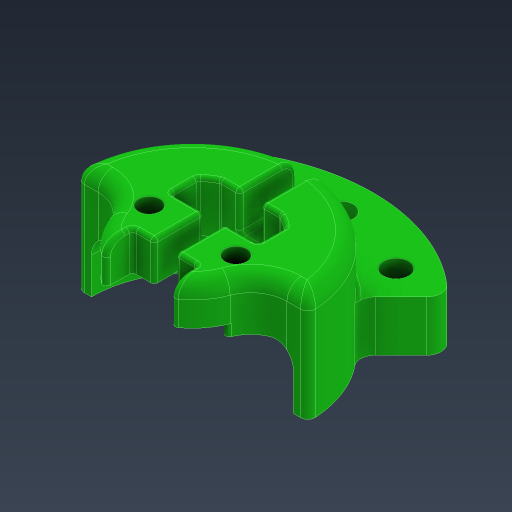
# Autodesk Inventor part: Крепление_энкодера
Saved by Autodesk Inventor 2023.2 (Build 272271030, 271C)
## iProperties
Created: 2026-01-03
Part Number: Крепление_энкодера
Material: Типовые
Document SubType Name: Modeling
Designer: Олег Коноваленко
Density: 1 g/cm^3
Appearance: Темно-зеленый
Author: Олег Коноваленко
Autodesk Inventor part; units mm, degrees
ref_plane "YZ Plane" through (0, 0, 0) normal (1, 0, 0) x (0, 1, 0)
ref_plane "XZ Plane" through (0, 0, 0) normal (0, 1, 0) x (-1, 0, 0)
ref_plane "XY Plane" through (0, 0, 0) normal (0, 0, 1) x (1, 0, 0)
sketch "Эскиз1" plane through (0, 0, 0) normal (0, 1, 0) x (-1, 0, 0)
  arc A0 (-14, 0) -> (14, 0) centre (0, 0) ccw
  arc A1 (-16, 0) -> (16, 0) centre (0, 0) ccw
  line L0 (-22.4, 0) -> (22.4, 0) projected
  dimension "d0" = 14
  dimension "d1" = 16
  constraints: 4 point on circle, 2 centre point, 2 point on line, 1 coincident
  measures "d0" radius of A0
  measures "d1" radius of A1
extrude "Выдавливание1" add sketch "Эскиз1" along normal blind 3 and the other way blind 5 contours A0 L0 A1
sketch "Эскиз2" plane through (0, 3, 0) normal (0, 1, 0) x (1, 0, 0)
  arc A0 (14, 0) -> (-14, 0) centre (0, 0) ccw projected
  circle A1 centre (0, 0) radius 9
  arc A2 (16, 0) -> (-16, 0) centre (0, 0) ccw projected
  line L0 (22.4, 0) -> (-22.4, 0) projected
  point P0 (-9, 0)
  point P1 (9, 0)
  dimension "d7" = 18
  constraints: 1 centre point, 1 coincident
  measures "d7" diameter of A1
extrude "Выдавливание2" add sketch "Эскиз2" along normal blind 7
fillet "Сопряжение2" radius 5 2 edges at (-9, 6.5, 0) (9, 6.5, 0)
fillet "Сопряжение3" radius 2 6 edges at (0, 10, -16) (10.242, 10, 0.8812) (14.5383, 10, 0) (-10.242, 10, 0.8812) (-14.5383, 10, 0) (0, 10, 9)
sketch "Эскиз3" plane through (0, 3, 0) normal (0, -1, 0) x (1, 0, 0)
  circle A0 centre (6, 0) radius 1.1 projected
  circle A1 centre (-6, 0) radius 1.1 projected
  circle A2 centre (-6, 0) radius 1.5
  circle A3 centre (6, 0) radius 1.5
  point P0 (0, 0)
  dimension "d12" = 3
  constraints: 2 centre point, 2 coincident, 1 equal radius
  measures "d12" diameter of A2
extrude "Выдавливание3" cut sketch "Эскиз3" against normal up to next contours A0 | A1 | A2 | A3
sketch "Эскиз4" plane through (0, 3, 0) normal (0, -1, 0) x (1, 0, 0)
  arc A0 (-7.5, -4.9749) -> (-4.1231, -8) centre (0, 0) ccw projected
  line L0 (4.1231, -8) -> (-4.1231, -8) projected
  arc A1 (4.1231, -8) -> (7.5, -4.9749) centre (0, 0) ccw projected
  line L1 (7.5, -4.9749) -> (7.5, 4.9749) projected
  arc A2 (7.5, 4.9749) -> (-7.5, 4.9749) centre (0, 0) ccw projected
  line L2 (-7.5, -4.9749) -> (-7.5, 4.9749) projected
extrude "Выдавливание4" cut sketch "Эскиз4" against normal blind 1.6
fillet "Сопряжение4" radius 0.5 2 edges at (-7.5, 3.8, 4.9749) (7.5, 3.8, 4.9749)
sketch "Эскиз5" plane through (0, -5, 0) normal (0, -1, 0) x (1, 0, 0)
  arc A0 (-17.6777, -17.6777) -> (17.6777, -17.6777) centre (0, 0) ccw
  line L0 (0, 5) -> (0, -30) construction
  line L1 (17.6777, -17.6777) -> (11.3137, -11.3137)
  arc A1 (-16, 0) -> (16, 0) centre (0, 0) ccw projected
  line L2 (-17.6777, -17.6777) -> (-11.3137, -11.3137)
  arc A2 (-14.4957, -14.4957) -> (14.4957, -14.4957) centre (0, 0) ccw construction
  circle A3 centre (10.6777, -17.4996) radius 1.75
  circle A4 centre (-10.6777, -17.4996) radius 1.75
  circle A5 centre (0, -20.5) radius 1.75
  point P0 (0, -25)
  dimension "d18" = 25
  dimension "d19" = 3.5
  dimension "d20" = 7
  dimension "d21" = 7
  constraints: 11 point on circle, 5 centre point, 4 end point, 2 coincident, 2 equal radius, 2 line through centre, 2 midpoint, 1 perpendicular, 1 point on line
  measures "d18" radius of A0
  measures "d19" diameter of A3
  measures "d20" horizontal distance of A3.centre L1.start
  measures "d21" horizontal distance of L2.start A4.centre
extrude "Выдавливание5" add sketch "Эскиз5" against normal blind 7
fillet "Сопряжение5" radius 2 4 edges at (11.3137, -1.5, -11.3137) (-11.3137, -1.5, -11.3137) (-17.6777, -1.5, -17.6777) (17.6777, -1.5, -17.6777)
sketch "Эскиз6" plane through (0, 4.6, 0) normal (0, -1, 0) x (1, 0, 0)
  line L0 (0, 15.8) -> (0, -31.8) construction
  line L1 (-4.5, 7.7942) -> (4.5, 7.7942) construction
  line L2 (4.5, 7.7942) -> (4.5, 3.7942)
  line L3 (4.5, 3.7942) -> (-4.5, 3.7942)
  line L4 (-4.5, 3.7942) -> (-4.5, 7.7942)
  line L5 (-4.5, 7.7942) -> (4.5, 3.7942) construction
  line L6 (4.5, 7.7942) -> (-4.5, 3.7942) construction
  arc A0 (8.4064, 3.2143) -> (-8.4064, 3.2143) centre (0, 0) ccw projected
  point P0 (0, 5.7942)
  point P1 (-4.5, 7.7942)
  dimension "d25" = 4
  dimension "d26" = 9
  constraints: 12 end point, 2 midpoint, 2 parallel, 1 horizontal, 1 perpendicular, 1 point on circle, 1 point on line
  measures "d25" distance of L1.end L2.end
  measures "d26" distance of L2.end L3.end
extrude "Выдавливание6" cut sketch "Эскиз6" against normal up to next
fillet "Сопряжение6" radius 0.5 9 edges at (-4.5, 9.4829, 7.0242) (-4.5, 10, 4.5781) (-4.5, 6.3, 7.7942) (4.5, 9.4829, 7.0242) (4.5, 10, 4.5781) (4.5, 6.3, 7.7942) (0, 10, 3.7942) (-4.5, 7.3, 3.7942) (4.5, 7.3, 3.7942)
sketch "Эскиз7" plane through (0, 3, 0) normal (0, -1, 0) x (1, 0, 0)
  line L0 (6, -8) -> (-6, -8)
  line L1 (-6, -8) -> (-6, -3)
  line L2 (-6, -3) -> (6, -3)
  line L3 (6, -3) -> (6, -8)
  line L4 (6, -8) -> (-6, -3) construction
  line L5 (-6, -8) -> (6, -3) construction
  line L6 (0, 13.9114) -> (0, -31.4852) construction
  line L7 (4.1231, -8) -> (-4.1231, -8) projected
  arc A0 (4.1231, -8) -> (7.5, -4.9749) centre (0, 0) ccw projected
  arc A1 (-7.5, -4.9749) -> (-4.1231, -8) centre (0, 0) ccw projected
  point P0 (0, 0)
  point P1 (0, -5.5)
  point P2 (0, -8)
  point P3 (-6, -6.7082)
  point P4 (6, -6.7082)
  dimension "d34" = 12
  dimension "d35" = 5
  constraints: 12 end point, 4 midpoint, 2 parallel, 1 horizontal, 1 perpendicular, 1 point on line
  measures "d34" distance of L1.end L2.end
  measures "d35" distance of L0.end L1.end
extrude "Выдавливание7" cut sketch "Эскиз7" against normal up to next contours L0 A1 L1 L2 L3 A0
sketch "Эскиз8" plane through (0, 10, 0) normal (0, 1, 0) x (1, 0, 0)
  line L0 (4, -3.7942) -> (-4, -3.7942) projected
  line L1 (-1.5, 16) -> (1.5, 16)
  line L2 (1.5, 16) -> (1.5, -3.7942)
  line L3 (1.5, -3.7942) -> (-1.5, -3.7942)
  line L4 (-1.5, -3.7942) -> (-1.5, 16)
  line L5 (0, 31.4852) -> (0, -13.9114) construction
  arc A0 (16, 0) -> (-16, 0) centre (0, 0) ccw projected
  point P0 (-1.5, -3.7942)
  point P1 (0, 16)
  dimension "d38" = 3
  constraints: 8 end point, 2 parallel, 2 point on line, 1 horizontal, 1 midpoint, 1 perpendicular, 1 point on circle
  measures "d38" distance between parallel lines of L2 L4
extrude "Выдавливание8" cut sketch "Эскиз8" against normal blind 5.4
fillet "Сопряжение7" radius 0.5 8 edges at (-1.5, 7.3, -3) (-1.5, 9.8536, 3.6478) (-1.5, 10, 0.1471) (-1.5, 7.05, 3.7942) (1.5, 9.8536, 3.6478) (1.5, 10, 0.1471) (1.5, 7.05, 3.7942) (1.5, 7.3, -3)
fillet "Сопряжение8" radius 0.5 10 edges at (-1.5, 9.4158, -15.3395) (-1.5, 6.3, -15.9295) (-1.5, 10, -10.9597) (1.5, 10, -10.9597) (1.5, 6.3, -15.9295) (1.5, 9.4158, -15.3395) (1.5, 4.6, -11.9648) (-1.5, 4.6, -11.9648) (0, 2, -16) (0, 4.6, -16)
fillet "Сопряжение9" radius 0.5 23 edges at (1.3536, 4.7464, -8) (0, 4.6, -8) (-1.3536, 4.7464, -8) (-1.5, 7.3, -8) (-1.6464, 9.8536, -8) (-3.0616, 10, -8) (1.6464, 9.8536, -8) (3.0616, 10, -8) (1.5, 7.3, -8) (5.1026, 10, -7.4137) (6, 10, -4.8541) (1.6464, 9.8536, -2.8536) (4, 10, -3) (-1.6464, 9.8536, -2.8536) (-4, 10, -3) (-5.1026, 10, -7.4137) (-6, 10, -4.8541) (-6, 7.3, -6.7082) (6, 7.3, -6.7082) (4.1231, 6.5, -8) (-4.1231, 6.5, -8) (-6, 7.3, -3) (6, 7.3, -3)
fillet "Сопряжение10" radius 3 1 edges at (0, 3, -14)
fillet "Сопряжение11" radius 1 4 edges at (-15.2198, 9.5702, -0.7612) (-16, 1.5, 0) (16, 1.5, 0) (15.2198, 9.5702, -0.7612)
